Dual Rocker Switch_v2 (Autodesk Fusion 360 design; units mm, degrees)
Autodesk Fusion 360 part; units mm, degrees
note: some values were not read from the file. Set by a fixed rule: which sketch regions a step uses.
sketch "Sketch1" plane through (0, 0, 0) normal (0, 1, 0) x (1, 0, 0)
  line L0 (10.9855, 12.8905) -> (-10.9855, 12.8905)
  line L1 (-10.9855, 12.8905) -> (-10.9855, -12.8905)
  line L2 (-10.9855, -12.8905) -> (10.9855, -12.8905)
  line L3 (10.9855, -12.8905) -> (10.9855, 12.8905)
  line L4 (10.9855, 12.8905) -> (-10.9855, -12.8905) construction
  line L5 (-10.9855, 12.8905) -> (10.9855, -12.8905) construction
  dimension "d1" = 21.971
  dimension "d2" = 25.781
  constraint horizontal L0
  constraint perpendicular L0 L1
  constraint parallel L0 L2
  constraint parallel L1 L3
  constraint coincident L4 origin
  constraint coincident L5 origin
  measures "d1" distance of L1.end L2.end
  measures "d2" distance of L0.start L2.end
extrude "Extrude1" add sketch "Sketch1" along normal blind 19.2786
sketch "Sketch2" plane through (0, 0, 0) normal (0, -1, 0) x (1, 0, 0)
  line L0 (10.9855, -12.8905) -> (10.9855, 12.8905)
  line L1 (10.9855, 12.8905) -> (-10.9855, 12.8905)
  line L2 (-10.9855, 12.8905) -> (-10.9855, -12.8905)
  line L3 (-10.9855, -12.8905) -> (10.9855, -12.8905)
  line L4 (12.192, -15.621) -> (-12.192, -15.621)
  line L5 (-12.192, -15.621) -> (-12.192, 15.621)
  line L6 (-12.192, 15.621) -> (12.192, 15.621)
  line L7 (12.192, 15.621) -> (12.192, -15.621)
  line L8 (12.192, -15.621) -> (-12.192, 15.621) construction
  line L9 (-12.192, -15.621) -> (12.192, 15.621) construction
  dimension "d5" = 24.384
  dimension "d6" = 31.242
  constraint horizontal L4
  constraint perpendicular L4 L5
  constraint parallel L4 L6
  constraint parallel L5 L7
  constraint coincident L8 origin
  constraint coincident L9 origin
  measures "d5" distance of L5.end L6.end
  measures "d6" distance of L4.end L5.end
extrude "Extrude2" add sketch "Sketch2" along normal blind 1.905 contours L0 L1 L2 L3 | L4 L5 L6 L7
sketch "Sketch3" plane through (0, -1.905, 0) normal (0, -1, 0) x (1, 0, 0)
  line L0 (12.192, 15.621) -> (-12.192, 15.621)
  line L1 (-12.192, 15.621) -> (-12.192, -15.621)
  line L2 (-12.192, -15.621) -> (12.192, -15.621)
  line L3 (12.192, -15.621) -> (12.192, 15.621)
  line L4 (-9.779, 12.0142) -> (-1.8288, 12.0142)
  line L5 (-1.8288, 12.0142) -> (-1.8288, -12.0142)
  line L6 (-1.8288, -12.0142) -> (-9.779, -12.0142)
  line L7 (-9.779, -12.0142) -> (-9.779, 12.0142)
  dimension "d9" = 3.6068
  dimension "d10" = 3.6068
  dimension "d11" = 2.413
  dimension "d12" = 7.9502
  constraint horizontal L4
  constraint vertical L5
  constraint horizontal L6
  constraint vertical L7
  measures "d9" distance of L0 L4
  measures "d10" distance of L2 L6
  measures "d11" distance of L1 L7
  measures "d12" distance of L4.start L4.end
ref_plane "WorkPlane1" through (-1.8288, -1.905, 0) normal (-1, 0, 0) x (0, 0, -1)
sketch "Sketch5" plane through (-1.8288, -1.905, 0) normal (-1, 0, 0) x (0, 1, 0)
  line L0 (0, -12.0142) -> (0, 12.0142)
  line L1 (0, 12.0142) -> (-4.3758, -7.048)
  arc A0 (-4.3758, -7.048) -> (0, -12.0142) centre (1.0537, -6.6748) ccw
  dimension "d14" = 19.558
  constraint coincident L0.end L1.start
  constraint coincident L0.start A0.end
  measures "d14" distance of L0.end L1.end
extrude "Extrude3" add sketch "Sketch5" along normal blind 7.9502
mirror "Mirror1" about plane through (0, 0, 0) normal (1, 0, 0) of "Extrude3"
equation "d10 = d9"
